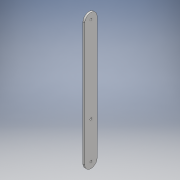
# Autodesk Inventor part: segment2
Saved by Autodesk Inventor 2017 (Build 210142000, 142)
## iProperties
Created: 2017-05-09
Part Number: segment2
Material: Ogólny
Document SubType Name: Modeling
Designer: Damian
Density: 1 g/cm^3
Appearance: Domyślna
Author: Damian
Autodesk Inventor part; units mm, degrees
ref_plane "YZ Plane" through (0, 0, 0) normal (1, 0, 0) x (0, 1, 0)
ref_plane "XZ Plane" through (0, 0, 0) normal (0, 1, 0) x (-1, 0, 0)
ref_plane "XY Plane" through (0, 0, 0) normal (0, 0, 1) x (1, 0, 0)
sketch "Szkic1" plane through (0, 0, 0) normal (1, 0, 0) x (0, 1, 0)
  line L0 (10, 0) -> (10, 0)
  line L1 (20, 10) -> (20, 210)
  line L2 (10, 220) -> (10, 220)
  line L3 (0, 210) -> (0, 10)
  arc A0 (20, 210) -> (10, 220) centre (10, 210) ccw
  arc A1 (10, 220) -> (0, 210) centre (10, 210) ccw
  arc A2 (10, 0) -> (20, 10) centre (10, 10) ccw
  arc A3 (0, 10) -> (10, 0) centre (10, 10) ccw
  circle A4 centre (10, 210) radius 1.6
  circle A5 centre (10, 70) radius 1.6
  circle A6 centre (10, 10) radius 1.6
  point P0 (0, 0)
  point P1 (20, 220)
  point P2 (0, 220)
  dimension "d0" = 20
  dimension "d1" = 10
  dimension "d2" = 200
  dimension "d3" = 60
  dimension "d4" = 3.2
  dimension "d5" = 3.2
  dimension "d6" = 3.2
  constraints: 8 end point, 8 point on circle, 8 tangent, 7 centre point, 6 point on line, 3 coincident, 3 equal radius, 2 parallel, 1 horizontal, 1 perpendicular
  measures "d0" distance of point (0, 220) point (20, 220)
  measures "d1" radius of A0
  measures "d2" distance of A2.centre A0.centre
  measures "d3" distance of point (10, 70) A2.centre
  measures "d4" diameter of A4
  measures "d5" diameter of A5
  measures "d6" diameter of A6
extrude "Wyciągnięcie proste1" add sketch "Szkic1" along normal blind 3
